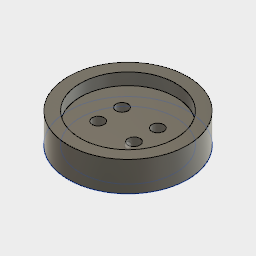
纽扣 (Autodesk Fusion 360 design; units mm, degrees)
Autodesk Fusion 360 part; units mm, degrees
sketch "草图1" plane through (0, 0, 0) normal (0, 1, 0) x (1, 0, 0)
  circle A0 centre (50, -35) radius 10
  circle A1 centre (50, -35) radius 8
  dimension "d1" = 2
extrude "拉伸1" add sketch "草图1" along normal blind 3 contours A1 makes body 1
extrude "拉伸2" add sketch "草图1" along normal blind 5 separate body makes body 2
cylinder "圆柱体基本要素1" add diameter 2 height 20 placed x (1, 0, 0) y (0, 0, -1) z (0, 1, 0) at (50, 0, 10) separate body makes body 3
move_body "移动1" bodies 3 to x (1, 0, 0) y (0, 1, 0) z (0, 0, 1) at (-2, 0, 21)
pattern_linear "R-阵列1" count 2 spacing 6 along (1, 0, 0) count 2 spacing 4 along (0, 0, 1) of bodies 3 makes body 4 at (54.995, 13.3333, 31.0996) makes body 5 at (47.1218, 6.6667, 34.5217) makes body 6 at (53.1218, 6.6667, 34.5217)
move_body "移动2" bodies 3 4 6 5 to x (1, 0, 0) y (0, 1, 0) z (0, 0, 1) at (-1, 0, 2)
combine "合并1" operation cut target body 1 tool bodies 4 5 6 3
